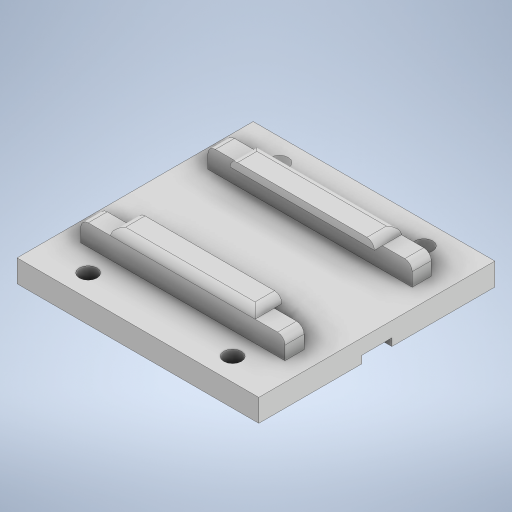
# Autodesk Inventor part: ESC_Mount
Saved by Autodesk Inventor 2024 (Build 280153000, 153)
## iProperties
Created: 2023-04-14
Part Number: ESC_Mount
Material: Generic
Document SubType Name: Modeling
Designer: richb366163
Density: 1 g/cm^3
Appearance: Default
Author: richb366163
Autodesk Inventor part; units mm, degrees
ref_plane "YZ Plane" through (0, 0, 0) normal (1, 0, 0) x (0, 1, 0)
ref_plane "XZ Plane" through (0, 0, 0) normal (0, 1, 0) x (-1, 0, 0)
ref_plane "XY Plane" through (0, 0, 0) normal (0, 0, 1) x (1, 0, 0)
sketch "Sketch1" plane through (0, 0, 0) normal (0, 1, 0) x (-1, 0, 0)
  line L0 (0, 0) -> (32.004, 0)
  line L1 (32.004, 0) -> (32.004, -17.0942)
  line L2 (32.004, -17.0942) -> (0, -17.0942)
  line L3 (0, -17.0942) -> (0, 0)
  line L4 (33.3375, -18.4277) -> (33.3375, 1.3335)
  line L5 (33.3375, 1.3335) -> (-1.3335, 1.3335)
  line L6 (-1.3335, 1.3335) -> (-1.3335, -18.4277)
  line L7 (-1.3335, -18.4277) -> (33.3375, -18.4277)
  line L8 (33.3375, 1.3335) -> (-1.3335, 1.3335)
  line L9 (-1.3335, 1.3335) -> (-1.3335, 11.4935)
  line L10 (-1.3335, 11.4935) -> (33.3375, 11.4935)
  line L11 (33.3375, 11.4935) -> (33.3375, 1.3335)
  line L12 (33.3375, -18.4277) -> (-1.3335, -18.4277)
  line L13 (-1.3335, -18.4277) -> (-1.3335, -28.575)
  line L14 (-1.3335, -28.575) -> (33.3375, -28.575)
  line L15 (33.3375, -28.575) -> (33.3375, -18.4277)
  line L16 (33.3375, 6.4135) -> (28.2575, 6.4135)
  circle A0 centre (28.2575, 7.6835) radius 1.5
  line L17 (33.3375, -8.5471) -> (26.9875, -8.5471)
  line L18 (16.002, 11.4935) -> (16.002, 8.6209)
  circle A1 centre (3.7465, 7.6835) radius 1.5
  circle A2 centre (28.2575, -24.7777) radius 1.5
  circle A3 centre (3.7465, -24.7777) radius 1.5
  line L19 (28.2575, 6.4135) -> (28.2575, 7.6835)
  line L20 (32.004, -8.5471) -> (35.179, -8.5471)
  line L21 (35.179, -8.5471) -> (33.3375, -8.5471)
  line L22 (33.3375, -8.5471) -> (33.3375, -28.575)
  line L23 (33.3375, -28.575) -> (35.179, -28.575)
  line L24 (35.179, -28.575) -> (35.179, -8.5471)
  line L25 (35.179, -8.5471) -> (33.3375, -8.5471)
  line L26 (33.3375, -8.5471) -> (33.3375, 11.4935)
  line L27 (33.3375, 11.4935) -> (35.179, 11.4935)
  line L28 (35.179, 11.4935) -> (35.179, -8.5471)
  line L29 (0, -8.5471) -> (-3.175, -8.5471)
  line L30 (-3.175, -8.5471) -> (-1.3335, -8.5471)
  line L31 (-1.3335, -8.5471) -> (-1.3335, 11.4935)
  line L32 (-1.3335, 11.4935) -> (-3.175, 11.4935)
  line L33 (-3.175, 11.4935) -> (-3.175, -8.5471)
  line L34 (-3.175, -8.5471) -> (-1.3335, -8.5471)
  line L35 (-1.3335, -8.5471) -> (-1.3335, -28.575)
  line L36 (-1.3335, -28.575) -> (-3.175, -28.575)
  line L37 (-3.175, -28.575) -> (-3.175, -8.5471)
  dimension "d0" = 32.004
  dimension "d1" = 17.0942
  dimension "d2" = 10.16
  dimension "d3" = 5.08
  dimension "d4" = 3
  dimension "d10" = 1.27
  dimension "d47" = 3.175
  dimension "d48" = 3.175
  constraints: 76 end point, 16 parallel, 10 horizontal, 8 perpendicular, 5 midpoint, 4 centre point, 2 collinear, 2 point on line, 2 vertical, 1 coincident, 1 symmetric about line, 6 other
  measures "d0" distance of L1.end L2.end
  measures "d1" distance of L0.end L1.end
  measures "d2" distance of L8.end L9.end
  measures "d3" distance of L16.start L16.end
  measures "d4" diameter of A0
  measures "d10" distance of L16.end L19.end
  measures "d47" distance of L20.start L20.end
  measures "d48" distance of L29.start L29.end
extrude "Extrusion1" add sketch "Sketch1" along normal blind 2.54 contours L3 L29 L6 L5 L4 L17 L1 L0 | L0 L1 L2 L3 | L3 L2 L1 L17 L4 L7 L6 L29 | L9 L10 L11 L5 | L7 L15 L14 L13
sketch "Sketch2" plane through (0, 2.54, 0) normal (0, 1, 0) x (1, 0, 0)
  line L0 (-33.3375, -11.4935) -> (1.3335, -11.4935) projected
  line L1 (1.3335, -11.4935) -> (1.3335, 28.575) projected
  line L2 (1.3335, 28.575) -> (-33.3375, 28.575) projected
  line L3 (-33.3375, 28.575) -> (-33.3375, -11.4935) projected
  circle A0 centre (-28.2575, -7.6835) radius 1.5 projected
  circle A1 centre (-3.7465, -7.6835) radius 1.5 projected
  circle A2 centre (-28.2575, 24.7777) radius 1.5 projected
  circle A3 centre (-3.7465, 24.7777) radius 1.5 projected
  line L4 (-33.3375, 28.575) -> (-33.3375, -11.4935) projected
  line L5 (1.3335, -11.4935) -> (-33.3375, -11.4935)
  line L6 (-33.3375, -11.4935) -> (-33.3375, -1.3335)
  line L7 (-33.3375, -1.3335) -> (1.3335, -1.3335)
  line L8 (1.3335, -1.3335) -> (1.3335, -11.4935)
  line L9 (1.3335, -11.4935) -> (1.3335, 28.575) projected
  line L10 (-33.3375, 28.575) -> (1.3335, 28.575)
  line L11 (1.3335, 28.575) -> (1.3335, 18.415)
  line L12 (1.3335, 18.415) -> (-33.3375, 18.415)
  line L13 (-33.3375, 18.415) -> (-33.3375, 28.575)
  line L14 (1.3335, 18.415) -> (-33.3375, 18.415)
  line L15 (-33.3375, 18.415) -> (-33.3375, 20.955)
  line L16 (-33.3375, 20.955) -> (1.3335, 20.955)
  line L17 (1.3335, 20.955) -> (1.3335, 18.415)
  line L18 (1.3335, -1.3335) -> (-33.3375, -1.3335)
  line L19 (-33.3375, -1.3335) -> (-33.3375, -3.8735)
  line L20 (-33.3375, -3.8735) -> (1.3335, -3.8735)
  line L21 (1.3335, -3.8735) -> (1.3335, -1.3335)
  line L22 (-33.3375, -1.3335) -> (1.3335, -1.3335)
  line L23 (1.3335, -1.3335) -> (1.3335, -0.635)
  line L24 (1.3335, -0.635) -> (-33.3375, -0.635)
  line L25 (-33.3375, -0.635) -> (-33.3375, -1.3335)
  line L26 (1.3335, 18.415) -> (-33.3375, 18.415)
  line L27 (-33.3375, 18.415) -> (-33.3375, 17.7165)
  line L28 (-33.3375, 17.7165) -> (1.3335, 17.7165)
  line L29 (1.3335, 17.7165) -> (1.3335, 18.415)
  point P0 (1.3335, 17.7165)
  point P1 (1.3335, 20.955)
  dimension "d34" = 10.16
  dimension "d35" = 10.16
  dimension "d36" = 2.54
  dimension "d37" = 2.54
  dimension "d38" = 0.6985
  dimension "d39" = 0.6985
  constraints: 48 end point, 12 parallel, 6 horizontal, 6 perpendicular, 6 point on line
  measures "d34" distance of L5.end L6.end
  measures "d35" distance of L10.end L11.end
  measures "d36" distance of L14.end L15.end
  measures "d37" distance of L19.end L18.end
  measures "d38" distance of L23.end L22.end
  measures "d39" distance of L27.end L26.end
extrude "Extrusion2" add sketch "Sketch2" along normal blind 3.556 contours L3 L7 L1 L20 | L3 L24 L1 L7 | L3 L12 L1 L28 | L3 L16 L1 L12
sketch "Sketch4" plane through (0, 0, 0) normal (0, -1, 0) x (1, 0, 0)
  line L0 (1.3335, 11.4935) -> (1.3335, -28.575) projected
  line L1 (1.3335, -8.5407) -> (-33.3375, -8.5407)
  line L2 (-33.3375, -28.575) -> (-33.3375, 11.4935) projected
  line L3 (1.3335, -11.0807) -> (-33.3375, -11.0807)
  line L4 (1.3335, -6.0007) -> (-33.3375, -6.0007)
  line L5 (-33.3375, 11.4935) -> (1.3335, 11.4935) projected
  line L6 (-33.3375, -28.575) -> (-33.3375, 11.4935) projected
  line L7 (1.3335, -28.575) -> (-33.3375, -28.575) projected
  line L8 (1.3335, 11.4935) -> (1.3335, -28.575) projected
  circle A0 centre (-28.2575, 7.6835) radius 1.5 projected
  circle A1 centre (-3.7465, 7.6835) radius 1.5 projected
  circle A2 centre (-28.2575, -24.7777) radius 1.5 projected
  circle A3 centre (-3.7465, -24.7777) radius 1.5 projected
  line L9 (1.3335, -6.0007) -> (11.5362, -6.0007)
  line L10 (11.5362, -6.0007) -> (11.5362, -11.0807)
  line L11 (11.5362, -11.0807) -> (1.3335, -11.0807)
  line L12 (1.3335, -11.0807) -> (1.3335, -6.0007)
  line L13 (-33.3375, -11.0807) -> (-46.0659, -11.0807)
  line L14 (-46.0659, -11.0807) -> (-46.0659, -6.0007)
  line L15 (-46.0659, -6.0007) -> (-33.3375, -6.0007)
  line L16 (-33.3375, -6.0007) -> (-33.3375, -11.0807)
  point P0 (0, 0)
  point P1 (1.3335, 1.3335)
  point P2 (1.3335, -18.4277)
  point P3 (-33.3375, -18.4277)
  point P4 (-33.3375, 1.3335)
  point P5 (1.3335, -18.4277)
  point P6 (1.3335, -11.0807)
  point P7 (-33.3375, -11.0807)
  point P8 (-33.3375, -18.4277)
  point P9 (-33.3375, 1.3335)
  point P10 (-33.3375, -6.0007)
  point P11 (1.3335, -6.0007)
  point P12 (1.3335, 1.3335)
  dimension "d16" = 2.54
  dimension "d17" = 2.54
  constraints: 22 end point, 6 parallel, 2 horizontal, 2 midpoint, 2 perpendicular, 1 point on line
  measures "d16" distance between parallel lines of L3 L1
  measures "d17" distance between parallel lines of L1 L4
extrude "Extrusion4" add sketch "Sketch4" along normal blind 1.27 contours L0 L4 L2 L5 | L0 L7 L2 L3
fillet "Fillet1" radius 6.35 8 edges at (1.3335, 1.27, 11.4935) (1.3335, -0.635, 11.4935) (1.3335, 1.27, -28.575) (1.3335, -0.635, -28.575) (-33.3375, 1.27, -28.575) (-33.3375, -0.635, -28.575) (-33.3375, 1.27, 11.4935) (-33.3375, -0.635, 11.4935)
fillet "Fillet3" radius 1.27 4 edges at (1.3335, 6.096, 2.2543) (1.3335, 6.096, -19.3357) (-33.3375, 6.096, -19.3357) (-33.3375, 6.096, 2.2543)
sketch "Sketch8" plane through (0, 6.096, 0) normal (0, 1, 0) x (1, 0, 0)
  line L0 (1.3335, -3.8735) -> (1.3335, -0.635) projected
  line L1 (0.0635, -0.635) -> (-32.0675, -0.635) projected
  line L2 (1.3335, -3.8735) -> (-3.7465, -3.8735)
  line L3 (-3.7465, -3.8735) -> (-3.7465, -0.635)
  line L4 (-3.7465, -0.635) -> (1.3335, -0.635)
  line L5 (1.3335, -0.635) -> (1.3335, -3.8735)
  line L6 (-33.3375, -3.8735) -> (-33.3375, -5.1435) projected
  line L7 (-33.3375, -3.8735) -> (-28.2575, -3.8735)
  line L8 (-28.2575, -3.8735) -> (-28.2575, -0.635)
  line L9 (-28.2575, -0.635) -> (-33.3375, -0.635)
  line L10 (-33.3375, -0.635) -> (-33.3375, -3.8735)
  line L11 (-28.2575, -3.8735) -> (-3.7465, -3.8735)
  line L12 (-3.7465, -3.8735) -> (-3.7465, 0.6985)
  line L13 (-3.7465, 0.6985) -> (-28.2575, 0.6985)
  line L14 (-28.2575, 0.6985) -> (-28.2575, -3.8735)
  line L15 (1.3335, -0.635) -> (1.3335, 17.7165) projected
  line L16 (1.3335, 8.5407) -> (-12.7, 8.5407)
  line L17 (-3.7465, 20.955) -> (-3.7465, 17.7165)
  line L18 (-28.2575, 20.955) -> (-3.7465, 20.955)
  line L19 (-3.7465, 20.955) -> (-3.7465, 16.383)
  line L20 (-3.7465, 16.383) -> (-28.2575, 16.383)
  line L21 (-28.2575, 16.383) -> (-28.2575, 20.955)
  point P0 (0, 0)
  point P1 (-3.7465, -0.635)
  point P2 (-28.2575, -0.635)
  dimension "d41" = 5.08
  dimension "d42" = 5.08
  dimension "d43" = 4.572
  constraints: 36 end point, 6 parallel, 6 symmetric about line, 4 horizontal, 4 point on line, 3 perpendicular, 1 midpoint
  measures "d41" distance of L3.end L4.end
  measures "d42" distance of L9.end L8.end
  measures "d43" distance of L12.end L11.end
extrude "Extrusion7" add sketch "Sketch8" along normal blind 1.27 contours L11 L8 L1 L3 | L1 L14 L13 L12 | L17 L19 L20 L21 L18
fillet "Fillet4" radius 1.27 6 edges at (-16.002, 7.366, -20.955) (-3.7465, 7.366, -18.669) (-28.2575, 7.366, -18.669) (-3.7465, 7.366, 1.5875) (-16.002, 7.366, 3.8735) (-28.2575, 7.366, 1.5875)
sketch "Sketch9" plane through (0, 2.54, 0) normal (0, 1, 0) x (1, 0, 0)
  line L0 (1.3335, 17.7165) -> (-33.3375, 17.7165) projected
  line L1 (-33.3375, 17.7165) -> (-33.3375, -0.635) projected
  line L2 (-33.3375, -0.635) -> (1.3335, -0.635) projected
  line L3 (1.3335, -0.635) -> (1.3335, 17.7165) projected
  line L4 (-5.0165, 28.575) -> (-26.9875, 28.575) projected
  line L5 (-33.3375, 8.5407) -> (-26.9875, 8.5407)
  line L6 (-26.9875, 8.5407) -> (-26.9875, 28.575)
  line L7 (-26.9875, 28.575) -> (-33.3375, 28.575)
  line L8 (-33.3375, 28.575) -> (-33.3375, 8.5407)
  line L9 (-33.3375, 28.575) -> (1.3335, 28.575)
  line L10 (1.3335, 28.575) -> (1.3335, -11.4935)
  line L11 (1.3335, -11.4935) -> (-33.3375, -11.4935)
  line L12 (-33.3375, -11.4935) -> (-33.3375, 28.575)
  line L13 (-33.3375, 8.5407) -> (-36.5125, 8.5407)
  line L14 (-36.5125, 8.5407) -> (-36.5125, 28.575)
  line L15 (-36.5125, 28.575) -> (-33.3375, 28.575)
  line L16 (-33.3375, 28.575) -> (-33.3375, 8.5407)
  line L17 (-36.5125, 8.5407) -> (-33.3375, 8.5407)
  line L18 (-33.3375, 8.5407) -> (-33.3375, -11.4935)
  line L19 (-33.3375, -11.4935) -> (-36.5125, -11.4935)
  line L20 (-36.5125, -11.4935) -> (-36.5125, 8.5407)
  line L21 (1.3335, -11.4935) -> (4.5085, -11.4935)
  line L22 (4.5085, -11.4935) -> (4.5085, 28.575)
  line L23 (4.5085, 28.575) -> (1.3335, 28.575)
  line L24 (1.3335, 28.575) -> (1.3335, -11.4935)
  arc A0 (-26.9875, 28.575) -> (-33.3375, 22.225) centre (-26.9875, 22.225) ccw projected
  line L25 (-33.3375, 22.225) -> (-33.3375, 20.955) projected
  line L26 (-33.3375, 20.955) -> (1.3335, 20.955) projected
  line L27 (1.3335, 20.955) -> (1.3335, 22.225) projected
  arc A1 (1.3335, 22.225) -> (-5.0165, 28.575) centre (-5.0165, 22.225) ccw projected
  line L28 (-5.0165, 28.575) -> (-26.9875, 28.575) projected
  circle A2 centre (-28.2575, 24.7777) radius 1.5 projected
  circle A3 centre (-3.7465, 24.7777) radius 1.5 projected
  arc A4 (-33.3375, -5.1435) -> (-26.9875, -11.4935) centre (-26.9875, -5.1435) ccw projected
  line L29 (-26.9875, -11.4935) -> (-5.0165, -11.4935) projected
  arc A5 (-5.0165, -11.4935) -> (1.3335, -5.1435) centre (-5.0165, -5.1435) ccw projected
  line L30 (1.3335, -5.1435) -> (1.3335, -3.8735) projected
  line L31 (1.3335, -3.8735) -> (-33.3375, -3.8735) projected
  line L32 (-33.3375, -3.8735) -> (-33.3375, -5.1435) projected
  circle A6 centre (-28.2575, -7.6835) radius 1.5 projected
  circle A7 centre (-3.7465, -7.6835) radius 1.5 projected
  point P0 (0, 0)
  point P1 (1.3335, -0.635)
  point P2 (1.3335, -5.1435)
  point P3 (-33.3375, -5.1437)
  point P4 (-33.3375, 8.5409)
  point P5 (-33.3375, 8.5409)
  dimension "d49" = 3.175
  dimension "d50" = 3.175
  constraints: 40 end point, 10 parallel, 5 horizontal, 5 perpendicular, 2 point on line, 1 midpoint
  measures "d49" distance of L14.end L15.end
  measures "d50" distance of L23.end L22.end
extrude "Extrusion8" add sketch "Sketch9" against normal blind 3.81 contours L10 L23 L22 L21 L3 | L1 L13 L14 L15 L8 | L12 L19 L20 L13 L1 | A1 L9 L10 | L10 L11 A5 | L8 L7 A0 | A4 L11 L12
sketch "Sketch11" plane through (0, -1.27, 0) normal (0, -1, 0) x (1, 0, 0)
  line L0 (1.3335, -6.0007) -> (1.3335, -11.0807) projected
  line L1 (1.3335, -6.0007) -> (1.3335, -11.0807)
  line L2 (1.3335, -11.0807) -> (4.5085, -11.0807)
  line L3 (4.5085, -11.0807) -> (4.5085, -6.0007)
  line L4 (4.5085, -6.0007) -> (1.3335, -6.0007)
  line L5 (-33.3375, -11.0807) -> (-33.3375, -6.0007) projected
  line L6 (-33.3375, -6.0007) -> (-33.3375, -11.0807)
  line L7 (-33.3375, -11.0807) -> (-36.5125, -11.0807)
  line L8 (-36.5125, -11.0807) -> (-36.5125, -6.0007)
  line L9 (-36.5125, -6.0007) -> (-33.3375, -6.0007)
  point P0 (0, 0)
  constraints: 16 end point, 6 equal length, 2 perpendicular
extrude "Extrusion9" cut sketch "Sketch11" against normal up to surface (1.27 mm away)
sketch "Sketch12" plane through (0, 2.54, 0) normal (0, 1, 0) x (1, 0, 0)
  line L0 (1.3335, -3.8735) -> (-33.3375, -3.8735) projected
  line L1 (-33.3375, -0.635) -> (-33.3375, -3.8735) projected
  line L2 (-33.3375, -0.635) -> (1.3335, -0.635) projected
  line L3 (1.3335, -3.8735) -> (1.3335, -0.635) projected
  line L4 (-36.5125, -11.4935) -> (4.5085, -11.4935) projected
  line L5 (4.5085, -11.4935) -> (4.5085, 28.575) projected
  line L6 (4.5085, 28.575) -> (-36.5125, 28.575) projected
  line L7 (-36.5125, 28.575) -> (-36.5125, -11.4935) projected
  circle A0 centre (-3.7465, -7.6835) radius 1.5 projected
  circle A1 centre (-28.2575, -7.6835) radius 1.5 projected
  line L8 (1.3335, 17.7165) -> (1.3335, 20.955) projected
  line L9 (1.3335, 17.7165) -> (-33.3375, 17.7165) projected
  line L10 (-33.3375, 20.955) -> (-33.3375, 17.7165) projected
  line L11 (-33.3375, 20.955) -> (1.3335, 20.955) projected
  circle A2 centre (-28.2575, 24.7777) radius 1.5 projected
  circle A3 centre (-3.7465, 24.7777) radius 1.5 projected
  line L12 (-26.9875, 16.383) -> (-26.9875, 19.685) projected
  line L13 (-26.9875, 16.383) -> (-5.0165, 16.383) projected
  line L14 (-5.0165, 19.685) -> (-5.0165, 16.383) projected
  line L15 (-26.9875, 19.685) -> (-5.0165, 19.685) projected
  line L16 (-5.0165, -2.6035) -> (-26.9875, -2.6035) projected
  line L17 (-5.0165, 0.6985) -> (-5.0165, -2.6035) projected
  line L18 (-5.0165, 0.6985) -> (-26.9875, 0.6985) projected
  line L19 (-26.9875, -2.6035) -> (-26.9875, 0.6985) projected
  point P0 (0, 0)
body "Solid1"
